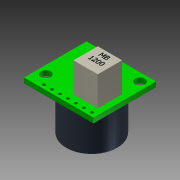
# Autodesk Inventor part: XL-MaxSonar MB1200
Saved by Autodesk Inventor 2012 (Build 160160000, 160)
## iProperties
Created: 2012-05-21
Part Number: XL-MaxSonar MB1200
Material: Default
Document SubType Name: Modeling
Designer: x02s
Density: 1 g/cm^3
Author: x02s
Autodesk Inventor part; units mm, degrees
ref_plane "YZ Plane" through (0, 0, 0) normal (1, 0, 0) x (0, 1, 0)
ref_plane "XZ Plane" through (0, 0, 0) normal (0, 1, 0) x (-1, 0, 0)
ref_plane "XY Plane" through (0, 0, 0) normal (0, 0, 1) x (1, 0, 0)
sketch "Sketch1" plane through (0, 0, 0) normal (0, 0, 1) x (1, 0, 0)
  line L0 (-11.05, 9.95) -> (11.05, 9.95)
  line L1 (11.05, 9.95) -> (11.05, -9.95)
  line L2 (11.05, -9.95) -> (-11.05, -9.95)
  line L3 (-11.05, -9.95) -> (-11.05, 9.95)
  circle A0 centre (-8.49, -5.55) radius 1.55
  circle A1 centre (8.51, 7.41) radius 1.55
  circle A2 centre (-5.89, -8.75) radius 0.5
  circle A3 centre (-3.35, -8.75) radius 0.5
  circle A4 centre (-0.81, -8.75) radius 0.5
  circle A5 centre (1.73, -8.75) radius 0.5
  circle A6 centre (4.27, -8.75) radius 0.5
  circle A7 centre (6.81, -8.75) radius 0.5
  circle A8 centre (9.35, -8.75) radius 0.5
  point P0 (0, 0)
  point P1 (-11.05, 0)
  point P2 (0, 9.95)
  dimension "d0" = 19.9
  dimension "d1" = 22.1
  dimension "d2" = 3.1
  dimension "d3" = 17
  dimension "d4" = 2.54
  dimension "d5" = 2.54
  dimension "d6" = 15.5
  dimension "d7" = 1
  dimension "d8" = 18.7
  dimension "d9" = 1.7
  dimension "d10" = 2.54
  dimension "d11" = 2.54
  dimension "d12" = 2.54
  dimension "d13" = 2.54
  dimension "d14" = 2.54
  dimension "d15" = 2.54
  constraints: 9 centre point, 8 end point, 7 equal radius, 7 horizontal alignment, 2 midpoint, 2 parallel, 1 horizontal, 1 perpendicular, 1 vertical alignment
  measures "d0" distance of L0.end L1.end
  measures "d1" distance of L0.start L0.end
  measures "d2" diameter of A0
  measures "d3" horizontal distance of A1.centre A0.centre
  measures "d4" distance from line of L1 A1.centre
  measures "d5" distance from line of A1.centre L0
  measures "d6" distance from line of L0 A0.centre
  measures "d7" diameter of A2
  measures "d8" distance from line of L0 A2.centre
  measures "d9" distance from line of A8.centre L1
  measures "d10" distance of A7.centre A8.centre
  measures "d11" distance of A6.centre A7.centre
  measures "d12" distance of A5.centre A6.centre
  measures "d13" distance of A4.centre A5.centre
  measures "d14" distance of A3.centre A4.centre
  measures "d15" distance of A2.centre A3.centre
extrude "Extrusion1" add sketch "Sketch1" along normal blind 1.6
sketch "Sketch2" plane through (0, 0, 1.6) normal (0, 0, 1) x (1, 0, 0)
  line L0 (1.45, 1.03) -> (9.17, 1.03)
  line L1 (9.17, 1.03) -> (9.17, -6.69)
  line L2 (9.17, -6.69) -> (1.45, -6.69)
  line L3 (1.45, -6.69) -> (1.45, 1.03)
  line L4 (-11.05, 9.95) -> (11.05, 9.95) projected
  line L5 (-11.05, -9.95) -> (-11.05, 9.95) projected
  point P0 (0, 0)
  dimension "d18" = 7.72
  dimension "d19" = 7.72
  dimension "d20" = 8.92
  dimension "d21" = 12.5
  constraints: 8 end point, 2 parallel, 1 horizontal, 1 perpendicular
  measures "d18" distance of L0.end L1.end
  measures "d19" distance of L0.start L0.end
  measures "d20" distance between parallel lines of L4 L0
  measures "d21" distance between parallel lines of L3 L5
extrude "Extrusion2" add sketch "Sketch2" along normal blind 9.36
sketch "Sketch3" plane through (0, 0, 0) normal (0, 0, -1) x (-1, 0, 0)
  circle A0 centre (0, 0.55) radius 8.2
  line L0 (-11.05, -9.95) -> (11.05, -9.95) projected
  point P0 (0, 0)
  dimension "d24" = 10.5
  dimension "d25" = 16.4
  constraints: 1 centre point, 1 vertical alignment
  measures "d24" distance from line of L0 A0.centre
  measures "d25" diameter of A0
extrude "Extrusion3" add sketch "Sketch3" along normal blind 13.64
sketch "Sketch5" plane through (0, 0.55, -13.64) normal (0, 0, -1) x (-1, 0, 0)
  circle A0 centre (0, 0) radius 8.2 projected
  line L0 (0, -6) -> (0, 6) construction
  line L1 (-6, 0) -> (6, 0) construction
  arc A1 (-1.5529, 5.7956) -> (-5.7956, 1.5529) centre (0, 0) ccw
  arc A2 (-5.7956, -1.5529) -> (-1.5529, -5.7956) centre (0, 0) ccw
  arc A3 (1.5529, -5.7956) -> (5.7956, -1.5529) centre (0, 0) ccw
  arc A4 (5.7956, 1.5529) -> (1.5529, 5.7956) centre (0, 0) ccw
  line L2 (1.9319, 0.5176) -> (2.8978, 0.7765)
  line L3 (4.3467, 1.1647) -> (5.7956, 1.5529)
  line L4 (1.9319, -0.5176) -> (2.8978, -0.7765)
  line L5 (4.3467, -1.1647) -> (5.7956, -1.5529)
  arc A5 (0.7765, -2.8978) -> (2.8978, -0.7765) centre (0, 0) ccw
  arc A6 (0.5176, -1.9319) -> (1.9319, -0.5176) centre (0, 0) ccw
  arc A7 (2.8978, 0.7765) -> (0.7765, 2.8978) centre (0, 0) ccw
  arc A8 (1.9319, 0.5176) -> (0.5176, 1.9319) centre (0, 0) ccw
  line L6 (-0.5176, 1.9319) -> (-0.7765, 2.8978)
  line L7 (-1.1647, 4.3467) -> (-1.5529, 5.7956)
  line L8 (-1.9319, 0.5176) -> (-2.8978, 0.7765)
  line L9 (-4.3467, 1.1647) -> (-5.7956, 1.5529)
  line L10 (0.5176, 1.9319) -> (0.7765, 2.8978)
  line L11 (1.1647, 4.3467) -> (1.5529, 5.7956)
  line L12 (0.5176, -1.9319) -> (0.7765, -2.8978)
  line L13 (1.1647, -4.3467) -> (1.5529, -5.7956)
  arc A9 (-0.7765, 2.8978) -> (-2.8978, 0.7765) centre (0, 0) ccw
  arc A10 (-2.8978, -0.7765) -> (-0.7765, -2.8978) centre (0, 0) ccw
  arc A11 (-0.5176, 1.9319) -> (-1.9319, 0.5176) centre (0, 0) ccw
  arc A12 (-1.9319, -0.5176) -> (-0.5176, -1.9319) centre (0, 0) ccw
  arc A13 (-1.1647, 4.3467) -> (-4.3467, 1.1647) centre (0, 0) ccw
  arc A14 (-4.3467, -1.1647) -> (-1.1647, -4.3467) centre (0, 0) ccw
  arc A15 (1.1647, -4.3467) -> (4.3467, -1.1647) centre (0, 0) ccw
  arc A16 (4.3467, 1.1647) -> (1.1647, 4.3467) centre (0, 0) ccw
  line L14 (-1.9319, -0.5176) -> (-2.8978, -0.7765)
  line L15 (-4.3467, -1.1647) -> (-5.7956, -1.5529)
  line L16 (-0.5176, -1.9319) -> (-0.7765, -2.8978)
  line L17 (-1.1647, -4.3467) -> (-1.5529, -5.7956)
  circle A17 centre (0, 0) radius 1
  point P0 (0, -0.55)
  dimension "d43" = 2
  dimension "d44" = 3
  dimension "d45" = 4.5
  dimension "d46" = 6
  dimension "d47" = 30
  dimension "d48" = 30
  dimension "d49" = 15
  dimension "d50" = 15
  dimension "d51" = 2
  constraints: 36 end point, 32 point on circle, 24 collinear, 17 centre point, 13 concentric, 6 point on line, 5 coincident, 3 midpoint, 1 perpendicular, 1 vertical
  measures "d43" radius of A8
  measures "d44" radius of A7
  measures "d45" radius of A16
  measures "d46" radius of A4
  measures "d47" angle of L13 L17
  measures "d48" angle of L3 L5
  measures "d49" angle of L1 L3
  measures "d50" angle of L13 L0
  measures "d51" diameter of A17
extrude "Extrusion4" cut sketch "Sketch5" against normal blind 10 contours L7 A13 L9 A1 | L15 A14 L17 A2 | L13 A15 L5 A3 | L3 A16 L11 A4 | A8 L10 A7 L2 | L4 A5 L12 A6 | A11 L8 A9 L6 | L14 A12 L16 A10 | A17
fillet "Fillet1" radius 0.5 1 edges at (8.2, 0.55, -13.64)
sketch "Sketch4" plane through (0, 0, 10.96) normal (0, 0, 1) x (1, 0, 0)
  line L0 (1.45, 1.03) -> (9.17, 1.03) projected
  line L1 (1.45, -6.69) -> (1.45, 1.03) projected
  line L2 (2.45, 0.03) -> (8.17, 0.03) construction
  line L3 (8.17, 0.03) -> (8.17, -5.69) construction
  line L4 (8.17, -5.69) -> (2.45, -5.69) construction
  line L5 (2.45, -5.69) -> (2.45, 0.03) construction
  line L6 (5.3453, -1.47) -> (5.1459, -1.47)
  line L7 (5.1459, -1.47) -> (5.1459, -0.1779)
  line L8 (5.1459, -0.1779) -> (4.7545, -1.0567)
  line L9 (4.7545, -1.0567) -> (4.6329, -1.0567)
  line L10 (4.6329, -1.0567) -> (4.2452, -0.1779)
  line L11 (4.2452, -0.1779) -> (4.2452, -1.47)
  line L12 (4.2452, -1.47) -> (4.0592, -1.47)
  line L13 (4.0592, -1.47) -> (4.0592, 0.03)
  line L14 (4.0592, 0.03) -> (4.3315, 0.03)
  line L15 (4.3315, 0.03) -> (4.7059, -0.8051)
  line L16 (4.7059, -0.8051) -> (5.0681, 0.03)
  line L17 (5.0681, 0.03) -> (5.3453, 0.03)
  line L18 (5.3453, 0.03) -> (5.3453, -1.47)
  spline S0 degree 2 poles (6.6666, -1.0093) (6.6666, -1.1211) (6.5815, -1.2925) (6.511, -1.3484) knots 0 0 0 1 2 2 2
  spline S1 degree 2 poles (6.511, -1.3484) (6.4259, -1.4141) (6.2326, -1.47) (6.0794, -1.47) knots 0 0 0 1 2 2 2
  line L19 (6.0794, -1.47) -> (5.6491, -1.47)
  line L20 (5.6491, -1.47) -> (5.6491, 0.03)
  line L21 (5.6491, 0.03) -> (6.0466, 0.03)
  spline S2 degree 2 poles (6.0466, 0.03) (6.2071, 0.03) (6.3675, 0.0093) (6.4405, -0.0308) knots 0 0 0 1 2 2 2
  spline S3 degree 2 poles (6.4405, -0.0308) (6.5219, -0.0733) (6.5961, -0.2131) (6.5961, -0.3079) knots 0 0 0 1 2 2 2
  spline S4 degree 2 poles (6.5961, -0.3079) (6.5961, -0.4137) (6.4842, -0.5814) (6.3858, -0.6288) knots 0 0 0 1 2 2 2
  line L22 (6.3858, -0.6288) -> (6.3858, -0.6361)
  spline S5 degree 2 poles (6.3858, -0.6361) (6.5195, -0.6726) (6.6666, -0.8659) (6.6666, -1.0093) knots 0 0 0 1 2 2 2
  spline S6 degree 2 poles (6.4587, -1.0178) (6.4587, -0.9327) (6.4101, -0.8233) (6.3371, -0.7844) knots 0 0 0 1 2 2 2
  spline S7 degree 2 poles (6.3371, -0.7844) (6.2897, -0.7601) (6.1779, -0.7455) (6.0746, -0.7455) knots 0 0 0 1 2 2 2
  line L23 (6.0746, -0.7455) -> (5.8485, -0.7455)
  line L24 (5.8485, -0.7455) -> (5.8485, -1.2998)
  line L25 (5.8485, -1.2998) -> (6.0102, -1.2998)
  spline S8 degree 2 poles (6.0102, -1.2998) (6.1414, -1.2998) (6.2922, -1.2755) (6.3505, -1.2366) knots 0 0 0 1 2 2 2
  spline S9 degree 2 poles (6.3505, -1.2366) (6.4064, -1.1965) (6.4587, -1.0968) (6.4587, -1.0178) knots 0 0 0 1 2 2 2
  spline S10 degree 2 poles (6.3882, -0.3359) (6.3882, -0.2824) (6.3517, -0.2022) (6.3116, -0.1791) knots 0 0 0 1 2 2 2
  spline S11 degree 2 poles (6.3116, -0.1791) (6.263, -0.1523) (6.1451, -0.1402) (6.0393, -0.1402) knots 0 0 0 1 2 2 2
  line L26 (6.0393, -0.1402) -> (5.8485, -0.1402)
  line L27 (5.8485, -0.1402) -> (5.8485, -0.579)
  line L28 (5.8485, -0.579) -> (6.0746, -0.579)
  spline S12 degree 2 poles (6.0746, -0.579) (6.1682, -0.579) (6.2569, -0.5595) (6.3043, -0.5292) knots 0 0 0 1 2 2 2
  spline S13 degree 2 poles (6.3043, -0.5292) (6.3505, -0.5) (6.3882, -0.4064) (6.3882, -0.3359) knots 0 0 0 1 2 2 2
  line L29 (4.0179, -3.9397) -> (3.2861, -3.9397)
  line L30 (3.2861, -3.9397) -> (3.2861, -3.7866)
  line L31 (3.2861, -3.7866) -> (3.5584, -3.7866)
  line L32 (3.5584, -3.7866) -> (3.5584, -2.7813)
  line L33 (3.5584, -2.7813) -> (3.2861, -2.7813)
  line L34 (3.2861, -2.7813) -> (3.2861, -2.6439)
  spline S14 degree 2 poles (3.2861, -2.6439) (3.4405, -2.6439) (3.5863, -2.5564) (3.5961, -2.4348) knots 0 0 0 1 2 2 2
  line L35 (3.5961, -2.4348) -> (3.7517, -2.4348)
  line L36 (3.7517, -2.4348) -> (3.7517, -3.7866)
  line L37 (3.7517, -3.7866) -> (4.0179, -3.7866)
  line L38 (4.0179, -3.7866) -> (4.0179, -3.9397)
  line L39 (5.2188, -3.9397) -> (4.2938, -3.9397)
  line L40 (4.2938, -3.9397) -> (4.2938, -3.727)
  spline S15 degree 2 poles (4.2938, -3.727) (4.3935, -3.6334) (4.5709, -3.4596) (4.656, -3.366) knots 0 0 0 1 2 2 2
  spline S16 degree 2 poles (4.656, -3.366) (4.8274, -3.1776) (4.9526, -2.9515) (4.9526, -2.8311) knots 0 0 0 1 2 2 2
  spline S17 degree 2 poles (4.9526, -2.8311) (4.9526, -2.7679) (4.9137, -2.6731) (4.8785, -2.6427) knots 0 0 0 1 2 2 2
  spline S18 degree 2 poles (4.8785, -2.6427) (4.8432, -2.6123) (4.7508, -2.5819) (4.6949, -2.5819) knots 0 0 0 1 2 2 2
  spline S19 degree 2 poles (4.6949, -2.5819) (4.6414, -2.5819) (4.532, -2.6087) (4.4822, -2.6293) knots 0 0 0 1 2 2 2
  spline S20 degree 2 poles (4.4822, -2.6293) (4.4397, -2.6464) (4.3606, -2.695) (4.3363, -2.712) knots 0 0 0 1 2 2 2
  line L41 (4.3363, -2.712) -> (4.3254, -2.712)
  line L42 (4.3254, -2.712) -> (4.3254, -2.4981)
  spline S21 degree 2 poles (4.3254, -2.4981) (4.3874, -2.4677) (4.6098, -2.4081) (4.7095, -2.4081) knots 0 0 0 1 2 2 2
  spline S22 degree 2 poles (4.7095, -2.4081) (4.9198, -2.4081) (5.1568, -2.6306) (5.1568, -2.8202) knots 0 0 0 1 2 2 2
  spline S23 degree 2 poles (5.1568, -2.8202) (5.1568, -2.9089) (5.1155, -3.0572) (5.079, -3.1204) knots 0 0 0 1 2 2 2
  spline S24 degree 2 poles (5.079, -3.1204) (5.0426, -3.1861) (4.9368, -3.3149) (4.8785, -3.3769) knots 0 0 0 1 2 2 2
  spline S25 degree 2 poles (4.8785, -3.3769) (4.7837, -3.4802) (4.5515, -3.7015) (4.4822, -3.7659) knots 0 0 0 1 2 2 2
  line L43 (4.4822, -3.7659) -> (5.2188, -3.7659)
  line L44 (5.2188, -3.7659) -> (5.2188, -3.9397)
  spline S26 degree 2 poles (6.3529, -3.1897) (6.3529, -3.5933) (6.1183, -3.9713) (5.874, -3.9713) knots 0 0 0 1 2 2 2
  spline S27 degree 2 poles (5.874, -3.9713) (5.626, -3.9713) (5.3939, -3.586) (5.3939, -3.1909) knots 0 0 0 1 2 2 2
  spline S28 degree 2 poles (5.3939, -3.1909) (5.3939, -2.7849) (5.6285, -2.4093) (5.874, -2.4093) knots 0 0 0 1 2 2 2
  spline S29 degree 2 poles (5.874, -2.4093) (6.1208, -2.4093) (6.3529, -2.7983) (6.3529, -3.1897) knots 0 0 0 1 2 2 2
  spline S30 degree 2 poles (6.0953, -3.6468) (6.1244, -3.5726) (6.1487, -3.3441) (6.1487, -3.1897) knots 0 0 0 1 2 2 2
  spline S31 degree 2 poles (6.1487, -3.1897) (6.1487, -3.0353) (6.1244, -2.808) (6.094, -2.7314) knots 0 0 0 1 2 2 2
  spline S32 degree 2 poles (6.094, -2.7314) (6.0636, -2.6549) (5.9579, -2.5759) (5.874, -2.5759) knots 0 0 0 1 2 2 2
  spline S33 degree 2 poles (5.874, -2.5759) (5.7901, -2.5759) (5.682, -2.6549) (5.6504, -2.7339) knots 0 0 0 1 2 2 2
  spline S34 degree 2 poles (5.6504, -2.7339) (5.62, -2.8105) (5.5981, -3.0438) (5.5981, -3.1909) knots 0 0 0 1 2 2 2
  spline S35 degree 2 poles (5.5981, -3.1909) (5.5981, -3.3489) (5.6175, -3.5605) (5.6491, -3.6431) knots 0 0 0 1 2 2 2
  spline S36 degree 2 poles (5.6491, -3.6431) (5.6783, -3.7209) (5.7865, -3.8048) (5.874, -3.8048) knots 0 0 0 1 2 2 2
  spline S37 degree 2 poles (5.874, -3.8048) (5.9567, -3.8048) (6.0649, -3.7258) (6.0953, -3.6468) knots 0 0 0 1 2 2 2
  spline S38 degree 2 poles (7.4786, -3.1897) (7.4786, -3.5933) (7.244, -3.9713) (6.9996, -3.9713) knots 0 0 0 1 2 2 2
  spline S39 degree 2 poles (6.9996, -3.9713) (6.7517, -3.9713) (6.5195, -3.586) (6.5195, -3.1909) knots 0 0 0 1 2 2 2
  spline S40 degree 2 poles (6.5195, -3.1909) (6.5195, -2.7849) (6.7541, -2.4093) (6.9996, -2.4093) knots 0 0 0 1 2 2 2
  spline S41 degree 2 poles (6.9996, -2.4093) (7.2464, -2.4093) (7.4786, -2.7983) (7.4786, -3.1897) knots 0 0 0 1 2 2 2
  spline S42 degree 2 poles (7.2209, -3.6468) (7.25, -3.5726) (7.2743, -3.3441) (7.2743, -3.1897) knots 0 0 0 1 2 2 2
  spline S43 degree 2 poles (7.2743, -3.1897) (7.2743, -3.0353) (7.25, -2.808) (7.2196, -2.7314) knots 0 0 0 1 2 2 2
  spline S44 degree 2 poles (7.2196, -2.7314) (7.1893, -2.6549) (7.0835, -2.5759) (6.9996, -2.5759) knots 0 0 0 1 2 2 2
  spline S45 degree 2 poles (6.9996, -2.5759) (6.9158, -2.5759) (6.8076, -2.6549) (6.776, -2.7339) knots 0 0 0 1 2 2 2
  spline S46 degree 2 poles (6.776, -2.7339) (6.7456, -2.8105) (6.7237, -3.0438) (6.7237, -3.1909) knots 0 0 0 1 2 2 2
  spline S47 degree 2 poles (6.7237, -3.1909) (6.7237, -3.3489) (6.7431, -3.5605) (6.7747, -3.6431) knots 0 0 0 1 2 2 2
  spline S48 degree 2 poles (6.7747, -3.6431) (6.8039, -3.7209) (6.9121, -3.8048) (6.9996, -3.8048) knots 0 0 0 1 2 2 2
  spline S49 degree 2 poles (6.9996, -3.8048) (7.0823, -3.8048) (7.1905, -3.7258) (7.2209, -3.6468) knots 0 0 0 1 2 2 2
  point P0 (0, 0)
  dimension "d29" = 1
  dimension "d30" = 1
  dimension "d31" = 1
  dimension "d32" = 1
  constraints: 2 other
  measures "d29" distance from line of L2.start L1
  measures "d30" distance from line of L0.end L3
  measures "d31" distance between parallel lines of L0 L2
  measures "d32" distance from line of L4 L1.start
emboss "Emboss1" sketch "Sketch4" operation add depth 0.1 direction (0, 0, -1)
equation "\"d11\" = d10"
equation "\"d12\" = d10"
equation "\"d13\" = d10"
equation "\"d14\" = d10"
equation "\"d15\" = d10"
equation "\"d19\" = d18"
equation "\"d48\" = d47"
equation "\"d49\" = 0.5 * d48"
equation "\"d50\" = 0.5 * d47"
equation "\"d30\" = d29"
equation "\"d31\" = d29"
equation "\"d32\" = d29"
equation "\"d40\" = 0.5 * d39"
equation "\"d41\" = d39"
equation "\"d42\" = d40"
equation "\"d39\" = 30deg"
body "Solid1"
